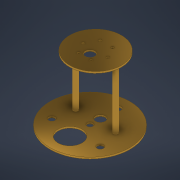
# Autodesk Inventor part: platform
Saved by Autodesk Inventor 2021 (Build 250183000, 183)
## iProperties
Created: 2020-12-23
Part Number: platform
Material: Steel, Mild
Document SubType Name: Modeling
Designer: Vikki
Density: 7.85 g/cm^3
Appearance: Brass - Polished
Mass: 141.387 g
Surface Area: 200.143 cm^2
Volume: 18.0111 cm^3
Author: Vikki
Autodesk Inventor part; units mm, degrees
ref_plane "YZ Plane" through (0, 0, 0) normal (1, 0, 0) x (0, 1, 0)
ref_plane "XZ Plane" through (0, 0, 0) normal (0, 1, 0) x (-1, 0, 0)
ref_plane "XY Plane" through (0, 0, 0) normal (0, 0, 1) x (1, 0, 0)
sketch "Sketch1" plane through (0, 0, 0) normal (0, 1, 0) x (-1, 0, 0)
  circle A0 centre (0, 0) radius 50
  circle A1 centre (0, -35) radius 3.75
  line L0 (0, -35) -> (0, 0) construction
  circle A2 centre (30.3109, 17.5) radius 3.75
  circle A3 centre (-30.3109, 17.5) radius 3.75
  circle A4 centre (0, 0) radius 3.75
  dimension "d0" = 100
  dimension "d1" = 35
  dimension "d2" = 7.5
  dimension "d5" = 360
  dimension "d9" = 7.5
  constraints: 5 centre point, 3 coincident, 2 end point, 1 vertical, 7 other
  measures "d0" diameter of A0
  measures "d1" distance of L0.start L0.end
  measures "d2" diameter of A1
  measures "d9" diameter of A4
extrude "Extrusion1" add sketch "Sketch1" along normal blind 2
sketch "Sketch2" plane through (0, 2, 0) normal (0, 1, 0) x (1, 0, 0)
  circle A0 centre (30.3109, -17.5) radius 3.75 projected
  circle A1 centre (30.3109, -17.5) radius 4
  point P0 (0, 0)
  dimension "d10" = 8
  constraints: 1 centre point, 1 coincident
  measures "d10" diameter of A1
extrude "Extrusion2" cut sketch "Sketch2" against normal blind 10
pattern_circular "Circular Pattern1" count 3 over 360 about axis through (0, 0, 0) along (0, 1, 0) of "Extrusion2"
sketch "Sketch7" plane through (0, 2, 0) normal (0, 1, 0) x (1, 0, 0)
  circle A0 centre (0, 13) radius 6
  point P0 (0, 0)
  dimension "d43" = 12
  dimension "d44" = 13
  constraints: 1 centre point, 1 vertical alignment
  measures "d43" diameter of A0
  measures "d44" distance of A0.centre point (0, 0)
extrude "Extrusion7" cut sketch "Sketch7" against normal up to surface (2 mm away)
sketch "Sketch9" plane through (0, 2, 0) normal (0, 1, 0) x (1, 0, 0)
  circle A0 centre (0, 7) radius 18.5 projected
  circle A1 centre (25, 7) radius 3
  circle A2 centre (-25, 7) radius 3
  point P0 (0, 0)
  dimension "d55" = 25
  dimension "d56" = 25
  dimension "d57" = 6
  constraints: 2 centre point, 2 horizontal alignment, 1 equal radius
  measures "d55" distance of A1.centre A0.centre
  measures "d56" distance of A2.centre A0.centre
  measures "d57" diameter of A1
extrude "Extrusion9" add sketch "Sketch9" along normal blind 75 contours A1 | A2
sketch "Sketch10" plane through (25, 77, -7) normal (0, 1, 0) x (1, 0, 0)
  circle A0 centre (-25, 0) radius 18.5 projected
  circle A1 centre (-25, 0) radius 32.5
  circle A2 centre (-25, -7) radius 6 projected
  circle A3 centre (-17.25, -13.4234) radius 1.6 projected
  circle A4 centre (-9.5, 0) radius 1.6 projected
  circle A5 centre (-17.25, 13.4234) radius 1.6 projected
  circle A6 centre (-32.75, 13.4234) radius 1.6 projected
  circle A7 centre (-40.5, 0) radius 1.6 projected
  circle A8 centre (-32.75, -13.4234) radius 1.6 projected
  point P0 (-25, -7)
  dimension "d60" = 65
  constraints: 1 centre point, 1 coincident
  measures "d60" diameter of A1
extrude "Extrusion10" add sketch "Sketch10" along normal blind 2 contours A0 | A1
sketch "Sketch11" plane through (0, 2, 0) normal (0, 1, 0) x (1, 0, 0)
  circle A0 centre (0, -25) radius 15
  point P0 (0, 0)
  dimension "d63" = 30
  dimension "d64" = 25
  constraints: 1 centre point, 1 vertical alignment
  measures "d63" diameter of A0
  measures "d64" distance of point (0, 0) A0.centre
extrude "Extrusion11" cut sketch "Sketch11" against normal up to surface (2 mm away)
equation "\"d56\" = d55"
body "Solid1"
